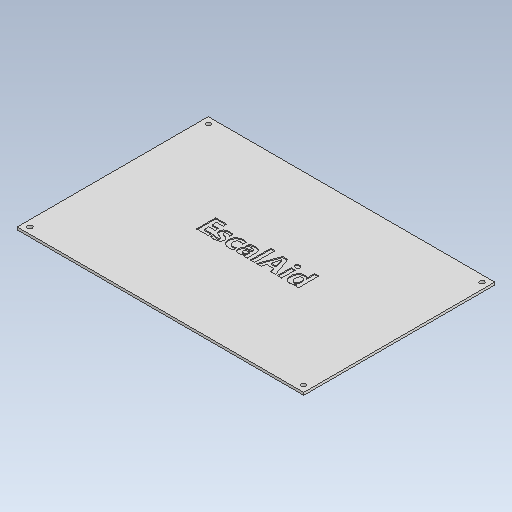
# Autodesk Inventor part: eboxlid
Saved by Autodesk Inventor 2025.2 (Build 292293000, 293)
## iProperties
Created: 2025-01-12
Part Number: eboxlid
Material: Generic
Document SubType Name: Modeling
Designer: email
Density: 1 g/cm^3
Appearance: Default
Author: email
Autodesk Inventor part; units mm, degrees
ref_plane "YZ Plane" through (0, 0, 0) normal (1, 0, 0) x (0, 1, 0)
ref_plane "XZ Plane" through (0, 0, 0) normal (0, 1, 0) x (-1, 0, 0)
ref_plane "XY Plane" through (0, 0, 0) normal (0, 0, 1) x (1, 0, 0)
sketch "Sketch1" plane through (0, 0, 0) normal (0, 1, 0) x (-1, 0, 0)
  line L0 (0, 0) -> (-225, 0)
  line L1 (-225, 0) -> (-225, -150)
  line L2 (-225, -150) -> (0, -150)
  line L3 (0, -150) -> (0, 0)
  circle A0 centre (-5, -145) radius 1.75
  circle A1 centre (-5, -5) radius 1.75
  circle A2 centre (-220, -5) radius 1.75
  circle A3 centre (-220, -145) radius 1.75
  dimension "d0" = 150
  dimension "d1" = 225
  dimension "d2" = 3.5
  dimension "d3" = 3.5
  dimension "d4" = 3.5
  dimension "d5" = 3.5
  dimension "d6" = 5
  dimension "d7" = 5
  dimension "d8" = 5
  dimension "d9" = 5
  dimension "d10" = 5
  dimension "d11" = 5
  dimension "d12" = 5
  dimension "d13" = 5
  constraints: 8 end point, 4 centre point, 2 parallel, 1 horizontal, 1 perpendicular
  measures "d0" distance between parallel lines of L0 L2
  measures "d1" distance of L1.end L2.end
  measures "d2" diameter of A0
  measures "d3" diameter of A3
  measures "d4" diameter of A1
  measures "d5" diameter of A2
  measures "d6" distance from line of L2 A0.centre
  measures "d7" distance from line of L3 A0.centre
  measures "d8" distance from line of L0 A1.centre
  measures "d9" distance from line of L3 A1.centre
  measures "d10" distance from line of L1 A2.centre
  measures "d11" distance from line of L0 A2.centre
  measures "d12" distance from line of L2 A3.centre
  measures "d13" distance from line of L1 A3.centre
extrude "Extrusion1" add sketch "Sketch1" along normal blind 2
sketch "Sketch2" plane through (0, 2, 0) normal (0, 1, 0) x (1, 0, 0)
  line L0 (70, 85) -> (155, 85) construction
  line L1 (155, 85) -> (155, 60) construction
  line L2 (155, 60) -> (70, 60) construction
  line L3 (70, 60) -> (70, 85) construction
  line L4 (0, 150) -> (0, 0) projected
  line L5 (225, 0) -> (225, 150) projected
  line L6 (225, 150) -> (0, 150) projected
  line L7 (0, 0) -> (225, 0) projected
  line L8 (80.7143, 69.1373) -> (71.7115, 69.1373)
  line L9 (71.7115, 69.1373) -> (71.7115, 84.1373)
  line L10 (71.7115, 84.1373) -> (80.3664, 84.1373)
  line L11 (80.3664, 84.1373) -> (80.3664, 81.3961)
  line L12 (80.3664, 81.3961) -> (75.0928, 81.3961)
  line L13 (75.0928, 81.3961) -> (75.0928, 78.0566)
  line L14 (75.0928, 78.0566) -> (80.0046, 78.0566)
  line L15 (80.0046, 78.0566) -> (80.0046, 75.3154)
  line L16 (80.0046, 75.3154) -> (75.0928, 75.3154)
  line L17 (75.0928, 75.3154) -> (75.0928, 71.8785)
  line L18 (75.0928, 71.8785) -> (80.7143, 71.8785)
  line L19 (80.7143, 71.8785) -> (80.7143, 69.1373)
  line L20 (82.1058, 69.4156) -> (82.1058, 72.1011)
  spline S0 degree 2 poles (82.1058, 72.1011) (82.9128, 71.6002) (84.5408, 71.1271) (85.2644, 71.1271) knots 0 0 0 1 2 2 2
  spline S1 degree 2 poles (85.2644, 71.1271) (86.141, 71.1271) (87.1568, 71.6002) (87.1568, 72.1011) knots 0 0 0 1 2 2 2
  spline S2 degree 2 poles (87.1568, 72.1011) (87.1568, 72.4072) (86.6976, 72.8247) (85.974, 73.1447) (85.1113, 73.3952) (84.7217, 73.5482) knots 0 0 0 1 2 3 4 4 4
  spline S3 degree 2 poles (84.7217, 73.5482) (84.0816, 73.7987) (83.1076, 74.3414) (82.4397, 75.0789) (82.1058, 76.039) (82.1058, 76.7069) knots 0 0 0 1 2 3 4 4 4
  spline S4 degree 2 poles (82.1058, 76.7069) (82.1058, 77.5974) (82.885, 78.9054) (84.1929, 79.7263) (85.8766, 80.116) (86.795, 80.116) knots 0 0 0 1 2 3 4 4 4
  spline S5 degree 2 poles (86.795, 80.116) (87.5046, 80.116) (88.9657, 79.8933) (89.6753, 79.6846) knots 0 0 0 1 2 2 2
  line L21 (89.6753, 79.6846) -> (89.6753, 77.1382)
  spline S6 degree 2 poles (89.6753, 77.1382) (89.0492, 77.5) (87.616, 77.8618) (86.9202, 77.8618) knots 0 0 0 1 2 2 2
  spline S7 degree 2 poles (86.9202, 77.8618) (86.6002, 77.8618) (86.0297, 77.7505) (85.5844, 77.5278) (85.334, 77.18) (85.334, 76.9573) knots 0 0 0 1 2 3 4 4 4
  spline S8 degree 2 poles (85.334, 76.9573) (85.334, 76.6651) (85.7096, 76.2477) (86.3219, 75.9555) (87.0594, 75.705) (87.4212, 75.5798) knots 0 0 0 1 2 3 4 4 4
  spline S9 degree 2 poles (87.4212, 75.5798) (88.0891, 75.3571) (89.1466, 74.8145) (89.9119, 74.077) (90.3293, 73.0891) (90.3293, 72.4072) knots 0 0 0 1 2 3 4 4 4
  spline S10 degree 2 poles (90.3293, 72.4072) (90.3293, 71.461) (89.4944, 70.1113) (88.1308, 69.2625) (86.3358, 68.8729) (85.3757, 68.8729) knots 0 0 0 1 2 3 4 4 4
  spline S11 degree 2 poles (85.3757, 68.8729) (83.6085, 68.8729) (82.1058, 69.4156) knots 0 0 0 1 1 1
  spline S12 degree 2 poles (100.3618, 69.5269) (99.2347, 68.8729) (97.1197, 68.8729) knots 0 0 0 1 1 1
  spline S13 degree 2 poles (97.1197, 68.8729) (94.6568, 68.8729) (91.5955, 71.8646) (91.5955, 74.2301) knots 0 0 0 1 2 2 2
  spline S14 degree 2 poles (91.5955, 74.2301) (91.5955, 76.9573) (94.8794, 80.116) (97.6206, 80.116) knots 0 0 0 1 2 2 2
  spline S15 degree 2 poles (97.6206, 80.116) (99.513, 80.116) (100.3618, 79.615) knots 0 0 0 1 1 1
  line L22 (100.3618, 79.615) -> (100.3618, 76.8043)
  spline S16 degree 2 poles (100.3618, 76.8043) (99.3182, 77.5835) (98.038, 77.5835) knots 0 0 0 1 1 1
  spline S17 degree 2 poles (98.038, 77.5835) (96.6187, 77.5835) (94.9629, 75.9137) (94.9629, 74.4527) knots 0 0 0 1 2 2 2
  spline S18 degree 2 poles (94.9629, 74.4527) (94.9629, 73.0334) (96.5492, 71.4054) (97.9406, 71.4054) knots 0 0 0 1 2 2 2
  spline S19 degree 2 poles (97.9406, 71.4054) (99.179, 71.4054) (100.3618, 72.1846) knots 0 0 0 1 1 1
  line L23 (100.3618, 72.1846) -> (100.3618, 69.5269)
  line L24 (111.4378, 69.1373) -> (108.3071, 69.1373)
  line L25 (108.3071, 69.1373) -> (108.3071, 70.6818)
  line L26 (108.3071, 70.6818) -> (108.2653, 70.6818)
  spline S20 degree 2 poles (108.2653, 70.6818) (107.18, 68.8729) (105.0649, 68.8729) knots 0 0 0 1 1 1
  spline S21 degree 2 poles (105.0649, 68.8729) (103.5065, 68.8729) (101.7254, 70.6401) (101.7254, 72.115) knots 0 0 0 1 2 2 2
  spline S22 degree 2 poles (101.7254, 72.115) (101.7254, 75.2319) (105.4128, 75.7189) knots 0 0 0 1 1 1
  line L27 (105.4128, 75.7189) -> (108.321, 76.1085)
  spline S23 degree 2 poles (108.321, 76.1085) (108.321, 77.8618) (106.4147, 77.8618) knots 0 0 0 1 1 1
  spline S24 degree 2 poles (106.4147, 77.8618) (104.5083, 77.8618) (102.7829, 76.7208) knots 0 0 0 1 1 1
  line L28 (102.7829, 76.7208) -> (102.7829, 79.2115)
  spline S25 degree 2 poles (102.7829, 79.2115) (103.4647, 79.5733) (105.872, 80.116) (106.846, 80.116) knots 0 0 0 1 2 2 2
  spline S26 degree 2 poles (106.846, 80.116) (111.4378, 80.116) (111.4378, 75.538) knots 0 0 0 1 1 1
  line L29 (111.4378, 75.538) -> (111.4378, 69.1373)
  line L30 (108.321, 73.4926) -> (108.321, 74.2161)
  line L31 (108.321, 74.2161) -> (106.3729, 73.9657)
  spline S27 degree 2 poles (106.3729, 73.9657) (104.7727, 73.757) (104.7727, 72.5046) knots 0 0 0 1 1 1
  spline S28 degree 2 poles (104.7727, 72.5046) (104.7727, 71.9481) (105.5519, 71.2245) (106.2199, 71.2245) knots 0 0 0 1 2 2 2
  spline S29 degree 2 poles (106.2199, 71.2245) (107.1521, 71.2245) (108.321, 72.5046) (108.321, 73.4926) knots 0 0 0 1 2 2 2
  line L32 (117.3655, 69.1373) -> (114.0538, 69.1373)
  line L33 (114.0538, 69.1373) -> (114.0538, 85)
  line L34 (114.0538, 85) -> (117.3655, 85)
  line L35 (117.3655, 85) -> (117.3655, 69.1373)
  line L36 (133.6735, 69.1373) -> (129.9861, 69.1373)
  line L37 (129.9861, 69.1373) -> (128.9147, 72.4768)
  line L38 (128.9147, 72.4768) -> (123.5853, 72.4768)
  line L39 (123.5853, 72.4768) -> (122.5278, 69.1373)
  line L40 (122.5278, 69.1373) -> (118.8683, 69.1373)
  line L41 (118.8683, 69.1373) -> (124.3228, 84.1373)
  line L42 (124.3228, 84.1373) -> (128.3302, 84.1373)
  line L43 (128.3302, 84.1373) -> (133.6735, 69.1373)
  line L44 (128.1494, 75.0649) -> (126.5353, 80.116)
  spline S30 degree 2 poles (126.5353, 80.116) (126.3544, 80.6725) (126.2848, 81.4657) knots 0 0 0 1 1 1
  line L45 (126.2848, 81.4657) -> (126.2013, 81.4657)
  spline S31 degree 2 poles (126.2013, 81.4657) (126.1456, 80.7978) (125.9369, 80.1577) knots 0 0 0 1 1 1
  line L46 (125.9369, 80.1577) -> (124.3089, 75.0649)
  line L47 (124.3089, 75.0649) -> (128.1494, 75.0649)
  line L48 (138.5297, 69.1373) -> (135.218, 69.1373)
  line L49 (135.218, 69.1373) -> (135.218, 79.8516)
  line L50 (135.218, 79.8516) -> (138.5297, 79.8516)
  line L51 (138.5297, 79.8516) -> (138.5297, 69.1373)
  spline S32 degree 2 poles (136.8878, 81.5492) (136.0529, 81.5492) (134.9814, 82.5371) (134.9814, 83.2607) knots 0 0 0 1 2 2 2
  spline S33 degree 2 poles (134.9814, 83.2607) (134.9814, 84.0121) (136.0529, 84.9443) (136.8878, 84.9443) knots 0 0 0 1 2 2 2
  spline S34 degree 2 poles (136.8878, 84.9443) (137.7365, 84.9443) (138.7941, 84.0121) (138.7941, 83.2607) knots 0 0 0 1 2 2 2
  spline S35 degree 2 poles (138.7941, 83.2607) (138.7941, 82.5093) (137.7365, 81.5492) (136.8878, 81.5492) knots 0 0 0 1 2 2 2
  line L52 (151.7904, 69.1373) -> (148.4926, 69.1373)
  line L53 (148.4926, 69.1373) -> (148.4926, 70.6122)
  line L54 (148.4926, 70.6122) -> (148.4508, 70.6122)
  spline S36 degree 2 poles (148.4508, 70.6122) (147.3237, 68.8729) (145.1252, 68.8729) knots 0 0 0 1 1 1
  spline S37 degree 2 poles (145.1252, 68.8729) (143.1215, 68.8729) (140.6725, 71.7115) (140.6725, 74.2579) knots 0 0 0 1 2 2 2
  spline S38 degree 2 poles (140.6725, 74.2579) (140.6725, 76.9156) (143.372, 80.116) (145.5566, 80.116) knots 0 0 0 1 2 2 2
  spline S39 degree 2 poles (145.5566, 80.116) (147.6299, 80.116) (148.4508, 78.6271) knots 0 0 0 1 1 1
  line L55 (148.4508, 78.6271) -> (148.4926, 78.6271)
  line L56 (148.4926, 78.6271) -> (148.4926, 85)
  line L57 (148.4926, 85) -> (151.7904, 85)
  line L58 (151.7904, 85) -> (151.7904, 69.1373)
  line L59 (148.5482, 74.3414) -> (148.5482, 75.1484)
  spline S40 degree 2 poles (148.5482, 75.1484) (148.5482, 76.2059) (147.3377, 77.5835) (146.3636, 77.5835) knots 0 0 0 1 2 2 2
  spline S41 degree 2 poles (146.3636, 77.5835) (145.2644, 77.5835) (144.0399, 75.8581) (144.0399, 74.3414) knots 0 0 0 1 2 2 2
  spline S42 degree 2 poles (144.0399, 74.3414) (144.0399, 72.936) (145.2226, 71.4054) (146.2801, 71.4054) knots 0 0 0 1 2 2 2
  spline S43 degree 2 poles (146.2801, 71.4054) (147.282, 71.4054) (148.5482, 73.0195) (148.5482, 74.3414) knots 0 0 0 1 2 2 2
  point P0 (155, 72.5)
  point P1 (112.5, 150)
  dimension "d16" = 70
  dimension "d17" = 70
  dimension "d18" = 65
  dimension "d19" = 60
  constraints: 2 midpoint, 2 other
  measures "d16" distance between parallel lines of L4 L3
  measures "d17" distance from line of L5 point (155, 72.5)
  measures "d18" distance from line of point (112.5, 150) L0
  measures "d19" distance between parallel lines of L7 L2
extrude "Extrusion2" cut sketch "Sketch2" against normal blind 0.75 contours L8 L9 L10 L11 L12 L13 L14 L15 L16 L17 L18 L19 | L20 S0 S1 S2 S3 S4 S5 L21 S6 S7 S8 S9 S10 S11 | S12 S13 S14 S15 L22 S16 S17 S18 S19 L23 | L24 L25 L26 S20 S21 S22 L27 S23 S24 L28 S25 S26 L29 | L32 L33 L34 L35 | L36 L37 L38 L39 L40 L41 L42 L43 | L48 L49 L50 L51 | S32 S33 S34 S35 | L52 L53 L54 S36 S37 S38 S39 L55 L56 L57 L58
body "Solid1"
